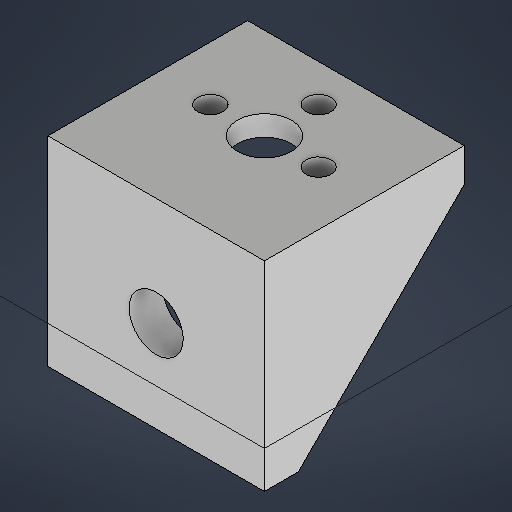
# Autodesk Inventor part: 000.001.004 - Уголок
Saved by Autodesk Inventor 2025 (Build 290162000, 162)
## iProperties
Created: 2022-02-27
Part Number: 000.001.004 - Уголок
Material: Типовые
Document SubType Name: Modeling
Designer: Petrov Ivan
Density: 1 g/cm^3
Appearance: По умолчанию
Author: Petrov Ivan
Autodesk Inventor part; units mm, degrees
ref_plane "YZ Plane" through (0, 0, 0) normal (1, 0, 0) x (0, 1, 0)
ref_plane "XZ Plane" through (0, 0, 0) normal (0, 1, 0) x (-1, 0, 0)
ref_plane "XY Plane" through (0, 0, 0) normal (0, 0, 1) x (1, 0, 0)
sketch "Эскиз1" plane through (0, 0, 0) normal (0, 1, 0) x (-1, 0, 0)
  circle A0 centre (8, 0) radius 1.85 projected
  circle A1 centre (0, 0) radius 4 projected
  circle A2 centre (0, 8) radius 1.85 projected
  circle A3 centre (-8, 0) radius 1.85 projected
  circle A4 centre (0, -8) radius 1.85 projected
  line L0 (-237.5, 16) -> (45.5, 16) projected
  line L1 (48, -13.5) -> (-240, -13.5) projected
  line L2 (12, -16) -> (-12, -16)
  line L3 (-12, -16) -> (-12, 16)
  line L4 (-12, 16) -> (12, 16)
  line L5 (12, 16) -> (12, -16)
  line L6 (12, -16) -> (-12, 16) construction
  line L7 (-12, -16) -> (12, 16) construction
  circle A5 centre (16, 0) radius 4 projected
  point P0 (-12, -13.5)
  point P1 (12, -13.5)
  constraints: 12 end point, 2 midpoint, 2 parallel, 1 horizontal, 1 perpendicular, 1 point on line, 1 tangent
extrude "Выдавливание1" add sketch "Эскиз1" against normal blind 5 contours A2 | L0 L5 L1 L3
sketch "Эскиз2" plane through (0, 0, 0) normal (0, 1, 0) x (1, 0, 0)
  line L0 (-12, -16) -> (-12, 13.5) projected
  line L1 (12, 13.5) -> (12, -16) projected
  line L2 (-12, -16) -> (12, -16)
  line L3 (12, -16) -> (12, -11)
  line L4 (12, -11) -> (-12, -11)
  line L5 (-12, -11) -> (-12, -16)
  point P0 (0, 0)
  point P1 (12, -16)
  point P2 (-12, -11)
  dimension "d2" = 5
  constraints: 8 end point, 2 parallel, 1 horizontal, 1 perpendicular, 1 point on line
  measures "d2" distance between parallel lines of L2 L4
extrude "Выдавливание2" add sketch "Эскиз2" against normal blind 29.5
sketch "Эскиз3" plane through (12, -5, 11) normal (0, 0, -1) x (-1, 0, 0)
  circle A0 centre (12, -11) radius 4 projected
  circle A1 centre (20, -11) radius 1.85 projected
  circle A2 centre (12, -19) radius 1.85 projected
  circle A3 centre (4, -11) radius 1.85 projected
  circle A4 centre (12, -3) radius 1.85 projected
  point P0 (12, 5)
extrude "Выдавливание3" cut sketch "Эскиз3" against normal through all contours A0
sketch "Эскиз4" plane through (-12, 0, -13.5) normal (-1, 0, 0) x (0, 0, 1)
  line L0 (24.5, -5) -> (24.5, -29.5) projected
  line L1 (24.5, -5) -> (0, -5) projected
  line L2 (24.5, -29.5) -> (0, -5)
  line L3 (0, 0) -> (29.5, 0) projected
  line L4 (0, 0) -> (0, -5) projected
  line L5 (24.5, -5) -> (0, -5) projected
  line L6 (24.5, -5) -> (24.5, -29.5) projected
  line L7 (29.5, -29.5) -> (24.5, -29.5) projected
  line L8 (29.5, 0) -> (29.5, -29.5) projected
  point P0 (13.5, 0)
  constraints: 2 end point
extrude "Выдавливание4" add sketch "Эскиз4" along normal blind 5
mirror "Зеркальное отражение1" about plane through (0, 0, 0) normal (1, 0, 0) of "Выдавливание4"
sketch "Эскиз5" plane through (0, -5, 0) normal (0, -1, 0) x (1, 0, 0)
  circle A0 centre (-8, 0) radius 1.85 projected
  circle A1 centre (-8, 0) radius 4
  circle A2 centre (0, 0) radius 4 projected
  line L0 (-8, 4) -> (0, 4)
  circle A3 centre (0, 0) radius 4 projected
  line L1 (-8, -4) -> (0, -4)
  point P0 (-4, 0)
  point P1 (0, -4)
  constraints: 4 end point, 4 point on circle, 2 tangent, 1 centre point, 1 coincident, 1 horizontal
extrude "Выдавливание5" cut sketch "Эскиз5" along normal blind 2 and the other way blind 2 contours A1 | A2 L1 A1 | A1 L0 A2
pattern_circular "Круговой массив1" count 3 over 180 about axis through (0, 0, 0) along (0, -1, 0) of "Выдавливание5"
fillet "Сопряжение1" radius 7.5 2 edges at (-4, -4, -4) (4, -4, -4)
move faces "Перенос1" translate (-1, 0, 0) faces at (17, -11.5, 4.5)
move faces "Перенос2" translate (1, 0, 0) faces at (-17, -11.5, 4.5)
